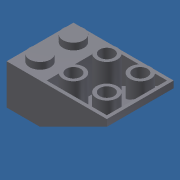
# Autodesk Inventor part: LEGO Brick 3747
Saved by Autodesk Inventor 2011 SP2 (Build 150309200, 309)
## iProperties
Created: 2011-09-28
Part Number: LEGO Brick 3747
Cost Center: 0 kg
Material: Steel
Document SubType Name: Modeling
Designer: BvH
Authority: 0 mm^3
Stock Number: =<Filenr>_<Document number>
Density: 7.85 g/cm^3
Company: Allseas Engineering BV
Subject: =<Title><TITLE 1_2> <TITLE 2_2>
Author: BvH
Act. Code: DW000
SaveDate: 2011-07-28
SaveTime: 18:32
FileName: Standard
TotalMass: 0 kg
TotalVolume: 0 mm^3
Autodesk Inventor part; units mm, degrees
ref_plane "YZ Plane" through (0, 0, 0) normal (1, 0, 0) x (0, 1, 0)
ref_plane "XY Plane" through (0, 0, 0) normal (0, 0, 1) x (1, 0, 0)
sketch "Sketch1" plane through (0, 0, 0) normal (0, 0, 1) x (1, 0, 0)
  line L0 (-12, 8) -> (12, 8)
  line L1 (12, 8) -> (12, -8)
  line L2 (12, -8) -> (-12, -8)
  line L3 (-12, -8) -> (-12, 8)
  line L4 (-12, -8) -> (12, 8) construction
  line L5 (-8, 4) -> (8, 4) construction
  line L6 (8, 4) -> (8, -4) construction
  line L7 (8, -4) -> (-8, -4) construction
  line L8 (-8, -4) -> (-8, 4) construction
  line L9 (-8, 4) -> (8, -4) construction
  circle A0 centre (-8, 4) radius 2.5
  circle A1 centre (0, 4) radius 2.5
  circle A2 centre (8, 4) radius 2.5
  circle A3 centre (8, -4) radius 2.5
  circle A4 centre (0, -4) radius 2.5
  circle A5 centre (-8, -4) radius 2.5
  line L10 (-4, 8) -> (-4, -8)
  point P0 (0, 0)
  point P1 (0, 0)
  dimension "d4" = 16
  dimension "d5" = 24
  dimension "d6" = 16
  dimension "d7" = 8
  dimension "d8" = 5
  dimension "d9" = 8
  constraints: 22 end point, 6 centre point, 5 coincident, 5 equal radius, 4 midpoint, 3 horizontal, 3 vertical, 2 parallel, 2 point on line, 1 perpendicular
  measures "d4" distance between parallel lines of L0 L2
  measures "d5" distance between parallel lines of L3 L1
  measures "d6" distance of L5.start L5.end
  measures "d7" distance of L5.end L6.end
  measures "d8" diameter of A0
  measures "d9" distance between parallel lines of L10 L3
extrude "Extrusion1" add sketch "Sketch1" along normal blind 9.6 contours L0 L10 L2 L3 | A0 | A5
extrude "Extrusion2" add sketch "Sketch1" along normal blind 9.6 separate body contours L0 L1 L2 L10 | A1 | A2 | A3 | A4
sketch "Sketch2" plane through (0, 0, 0) normal (0, 1, 0) x (-1, 0, 0)
  line L0 (-12, 0) -> (-12, 9.6) construction
  line L1 (4, 0) -> (4, 9.6) construction
  line L2 (4, 0) -> (-12, 8)
  dimension "d14" = 1.6
  constraints: 2 end point, 1 point on line
  measures "d14" distance of L2.end L0.end
ref_plane "Work Plane1" through (-4, 0, 0) normal (-0.4472136, 0, 0.8944272) x (0.8944272, 0, 0.4472136)
extrude "Extrusion3" add sketch "Sketch1" along normal blind 11.2 separate body contours A1 | A2 | A3 | A4
extrude "Extrusion4" add sketch "Sketch1" along normal blind 11.2 separate body contours A0 | A5
split "Split1" plane through (-4, 0, 0) removes the side toward (0.4472136, 0, -0.8944272)
split "Split2" plane through (-4, 0, 0) removes the side toward (0.4472136, 0, -0.8944272)
shell "Shell1" thickness 0.8 removed faces 1 at (6.6667, -2.6667, 9.6) bodies 2
shell "Shell2" thickness 0.8 removed faces 4 at (-0.1004, 4.8273, 11.2) at (7.0612, 3.6127, 11.2) at (7.7045, -3.2208, 11.2) at (-0.1004, -3.2689, 11.2) bodies 3
combine bodies "Combine1" operation type add bodies to combine 1 2 3 4
sketch "Sketch3" plane through (-4, 8, 0) normal (0, 0, -1) x (-1, 0, 0)
  circle A0 centre (4, -12) radius 2.5 construction
  circle A1 centre (4, -4) radius 2.5 construction
  line L0 (6.5, -14.5) -> (1.5, -14.5)
  line L1 (1.5, -14.5) -> (1.5, -1.5)
  line L2 (1.5, -1.5) -> (6.5, -1.5)
  line L3 (6.5, -1.5) -> (6.5, -14.5)
  constraints: 8 end point, 4 tangent, 2 parallel, 1 horizontal, 1 perpendicular
extrude "Extrusion5" cut sketch "Sketch3" against normal blind 1.6 bodies 1
body "Solid1"
